patin v8 (Autodesk Fusion 360 design; units mm, degrees)
Autodesk Fusion 360 part; units mm, degrees
sketch "Sketch1" plane through (0, 0, 0) normal (0, 0, 1) x (1, 0, 0)
  line L0 (0, 0) -> (20, 0)
  line L1 (20, 0) -> (20, 50)
  line L2 (20, 50) -> (0, 50)
  line L3 (0, 50) -> (0, 0)
  line L4 (20, 25) -> (0, 25) construction
  line L5 (12.5, 42.5) -> (12.5, 7.5) construction
  circle A0 centre (12.5, 7.5) radius 1.75
  circle A1 centre (12.5, 42.5) radius 1.75
  dimension "d1" = 50
  dimension "d2" = 20
  dimension "d3" = 35
  dimension "d4" = 3.5
  dimension "d5" = 12.5
  constraint horizontal L0
  constraint vertical L1
  constraint horizontal L2
  constraint vertical L3
  constraint coincident L0.start L3.end
  constraint midpoint L1 L0.start
  constraint midpoint L3 L0.start
  constraint perpendicular L4 L5
  constraint equal A0 A1
  measures "d4" diameter of A1
  measures "d5" distance of L3 L5
extrude "Extrude1" add sketch "Sketch1" along normal blind 2
sketch "Sketch2" plane through (0, 0, 0) normal (-1, 0, 0) x (0, -1, 0)
  line L0 (-50, 0) -> (0, 0)
  line L1 (0, 0) -> (0, 2)
  line L2 (0, 2) -> (-50, 2)
  line L3 (-50, 2) -> (-50, 0)
  line L4 (-50, 0) -> (-50, -15) construction
  line L5 (0, 0) -> (0, -15) construction
  line L6 (-25, 0) -> (-25, -30) construction
  line L7 (0, 2) -> (10, -15)
  line L8 (-50, 2) -> (-60, -15)
  line L9 (-60, -15) -> (-50, -15) construction
  line L10 (0, -15) -> (10, -15) construction
  line L11 (-3.8235, 0) -> (5, -15)
  line L12 (-46.1765, 0) -> (-55, -15)
  line L13 (5, -15) -> (10, -15)
  line L14 (-3.8235, 0) -> (0, 2)
  line L15 (-46.1765, 0) -> (-50, 2)
  line L16 (-60, -15) -> (-55, -15)
  dimension "d8" = 15
  dimension "d10" = 70
  dimension "d11" = 5
  dimension "d12" = 5
  constraint coincident L0.end L1.start
  constraint perpendicular L0 L4
  constraint perpendicular L0 L5
  constraint equal L4 L5
  constraint midpoint L0 L1.start
  constraint perpendicular L0 L6
  constraint perpendicular L4 L9
  constraint perpendicular L5 L10
  constraint coincident L0 L1.start
  constraint coincident L10 L0.end
  constraint parallel L7 L11
  constraint coincident L9 L0.end
  constraint parallel L8 L12
extrude "Extrude2" add sketch "Sketch2" against normal blind 20 contours L0 L3 L8 L12 L16 | L0 L1 L7 L11 L13
sketch "Sketch3" plane through (0, 0, 0) normal (-1, 0, 0) x (0, -1, 0)
  line L0 (-46.1765, 0) -> (-3.8235, 0)
  line L1 (-3.8235, 0) -> (5, -15)
  line L2 (5, -15) -> (10, -15)
  line L3 (10, -15) -> (0, 2)
  line L4 (0, 2) -> (-50, 2)
  line L5 (-50, 2) -> (-60, -15)
  line L6 (-60, -15) -> (-55, -15)
  line L7 (-55, -15) -> (-46.1765, 0)
  line L8 (-55, -15) -> (15, -15)
  line L9 (15, -15) -> (15, -12)
  line L10 (15, -12) -> (-55, -12)
  line L11 (-55, -12) -> (-55, -15)
  dimension "d15" = 3
  constraint horizontal L8
  constraint vertical L9
  constraint horizontal L10
  constraint vertical L11
extrude "Extrude3" add sketch "Sketch3" against normal blind 20 contours L1 L7 L8 L10
sketch "Sketch6" plane through (0, 0, 0) normal (-1, 0, 0) x (0, -1, 0)
  line L0 (-60, -15) -> (10, -15)
  line L1 (10, -15) -> (0, 2)
  line L2 (0, 2) -> (-50, 2)
  line L3 (-50, 2) -> (-60, -15)
  line L4 (3.2353, -12) -> (-53.2353, -12)
  line L5 (-53.2353, -12) -> (-46.1765, 0)
  line L6 (-46.1765, 0) -> (-3.8235, 0)
  line L7 (-3.8235, 0) -> (3.2353, -12)
  line L8 (-25, 2) -> (-25, -15) construction
  line L9 (-75, -12) -> (25, -12)
  line L10 (25, -12) -> (25, -15)
  line L11 (25, -15) -> (-75, -15)
  line L12 (-75, -15) -> (-75, -12)
  dimension "d36" = 100
  constraint midpoint L2 origin
  constraint midpoint L0 origin
  constraint horizontal L9
  constraint vertical L10
  constraint horizontal L11
  constraint vertical L12
  constraint collinear L4 L9
  constraint collinear L0 L11
extrude "Extrude5" add sketch "Sketch6" against normal blind 10 contours L0 L1 L3 L4 L9 L11 | L3 L9 L11 L12 | L1 L9 L10 L11
sketch "Sketch4" plane through (0, 0, -15) normal (0, 0, -1) x (1, 0, 0)
  line L0 (0, 25) -> (0, -75)
  line L1 (10, -60) -> (20, -60)
  line L2 (20, -60) -> (20, 10)
  line L3 (20, 10) -> (10, 10)
  line L4 (20, -25) -> (0, -25) construction
  line L5 (10, 20) -> (30, 20)
  line L6 (30, 20) -> (30, -70)
  line L7 (30, -70) -> (10, -70)
  line L8 (10, -70) -> (10, 20)
  line L9 (10, 20) -> (30, -70) construction
  line L10 (30, 20) -> (10, -70) construction
  line L11 (10, 10) -> (10, 25)
  line L12 (10, 25) -> (0, 25)
  line L13 (0, -75) -> (10, -75)
  line L14 (10, -75) -> (10, -60)
  dimension "d18" = 90
  dimension "d19" = 20
  constraint midpoint L2 origin
  constraint midpoint L0 origin
  constraint perpendicular L5 L6
  constraint parallel L5 L7
  constraint parallel L6 L8
  constraint horizontal L5
  constraint coincident L9 origin
  constraint coincident L10 origin
  measures "d18" distance of origin
extrude "Extrude4" cut sketch "Sketch4" against normal blind 16 contours L1 L2 L3 L5 L6 L7 L8 L11 L14 | L1 L2 L3 L8
chamfer "Chamfer2" distance 3 angle 45 2 edges at (5, 75, -15) (5, -25, -15)
fillet "Fillet3" radius 20 2 edges at (5, 72, -15) (5, -22, -15)
chamfer "Chamfer3" distance 1 angle 45 1 edges at (10, 25, 0)
fillet "Fillet4" radius 10 2 edges at (10, 48.0882, 1) (10, 1.9118, 1)
equation "d5 = 5 mm + 7.5 mm"
